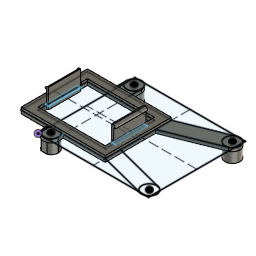
Eris LCD Mount Pi Attachment v2 (Autodesk Fusion 360 design; units mm, degrees)
Autodesk Fusion 360 part; units mm, degrees
sketch "Sketch1" plane through (0, 0, 0) normal (0, 0, 1) x (1, 0, 0)
  line L0 (0, 0) -> (65, 0)
  line L1 (65, 0) -> (65, 57)
  line L2 (65, 57) -> (0, 57)
  line L3 (0, 57) -> (0, 0)
  line L4 (-17, 7) -> (32.5, 7)
  line L5 (32.5, 7) -> (32.5, 46)
  line L6 (32.5, 46) -> (-17, 46)
  line L7 (-17, 46) -> (-17, 7)
  line L8 (7.75, 46) -> (7.75, 7) construction
  line L9 (-17, 26.5) -> (32.5, 26.5) construction
  line L10 (-12, 12) -> (27.5, 12)
  line L11 (27.5, 12) -> (27.5, 41)
  line L12 (27.5, 41) -> (-12, 41)
  line L13 (-12, 41) -> (-12, 12)
  line L14 (-12, 26.5) -> (-11, 26.5) construction
  line L15 (-11, 26.5) -> (-11, 36)
  line L16 (-11, 36) -> (-12, 36)
  line L17 (-12, 36) -> (-12, 26.5) construction
  line L18 (-11, 26.5) -> (-12, 26.5) construction
  line L19 (-12, 26.5) -> (-12, 17) construction
  line L20 (-12, 17) -> (-11, 17)
  line L21 (-11, 17) -> (-11, 26.5)
  line L22 (27.5, 36) -> (26.25, 36)
  line L23 (26.25, 36) -> (26.25, 26.5)
  line L24 (26.25, 26.5) -> (27.5, 26.5) construction
  line L25 (27.5, 26.5) -> (27.5, 36) construction
  line L26 (27.5, 26.5) -> (26.25, 26.5) construction
  line L27 (26.25, 26.5) -> (26.25, 17)
  line L28 (26.25, 17) -> (27.5, 17)
  line L29 (27.5, 17) -> (27.5, 26.5) construction
  line L30 (-12, 36) -> (-13, 36)
  line L31 (-13, 36) -> (-13, 17)
  line L32 (-13, 17) -> (-12, 17)
  line L33 (-12, 17) -> (-12, 36)
  line L34 (27.5, 36) -> (28.5, 36)
  line L35 (28.5, 36) -> (28.5, 17)
  line L36 (28.5, 17) -> (27.5, 17)
  line L37 (27.5, 17) -> (27.5, 36)
  line L38 (32.5, 57) -> (32.5, 0) construction
  line L39 (65, 28.5) -> (0, 28.5) construction
  circle A0 centre (3.5, 53) radius 1.35
  circle A1 centre (61.5, 53) radius 1.35
  circle A2 centre (61.5, 4) radius 1.35
  circle A3 centre (3.5, 4) radius 1.35
  circle A4 centre (3.5, 53) radius 4.35
  circle A5 centre (61.5, 53) radius 4.35
  circle A6 centre (3.5, 4) radius 4.35
  circle A7 centre (61.5, 4) radius 4.35
  line L40 (7.75, 46) -> (7.8496, 52.9376)
  line L41 (-0.8496, 53.0624) -> (-0.9509, 46)
  line L42 (7.8496, 4.0624) -> (7.75, 7)
  line L43 (32.5, 7) -> (60.4118, -0.2117)
  line L44 (32.5, 46) -> (59.8736, 57.0345)
  line L45 (32.5, 15.9857) -> (62.5882, 8.2117)
  line L46 (32.5, 36.6197) -> (63.1264, 48.9655)
  line L47 (-0.85, 4) -> (-0.85, 7)
  dimension "d1" = 65
  dimension "d2" = 57
  dimension "d3" = 17
  dimension "d5" = 49.5
  dimension "d6" = 39
  dimension "d7" = 7
  dimension "d8" = -5
  dimension "d13" = 1
  dimension "d21" = 2.7
  dimension "d22" = 2.7
  dimension "d23" = 2.7
  dimension "d24" = 2.7
  dimension "d26" = 29
  dimension "d27" = 29
  dimension "d28" = 29
  dimension "d29" = 29
  dimension "d30" = 24.5
  dimension "d31" = 24.5
  dimension "d32" = 24.5
  dimension "d33" = 24.5
  dimension "d34" = 3
  dimension "d35" = 3
  dimension "d36" = 3
  dimension "d37" = 3
  constraint horizontal L0
  constraint vertical L1
  constraint horizontal L2
  constraint vertical L3
  constraint coincident L0.start L3.end
  constraint horizontal L4
  constraint vertical L5
  constraint horizontal L6
  constraint vertical L7
  constraint midpoint L6 L8.start
  constraint midpoint L4 L8.end
  constraint midpoint L7 L9.start
  constraint midpoint L5 L9.end
  constraint midpoint L13 L14.start
  constraint coincident L13 L19.end
  constraint horizontal L14
  constraint vertical L15
  constraint horizontal L16
  constraint vertical L17
  constraint horizontal L18
  constraint vertical L19
  constraint horizontal L20
  constraint vertical L21
  constraint horizontal L22
  constraint vertical L23
  constraint horizontal L24
  constraint vertical L25
  constraint horizontal L26
  constraint vertical L27
  constraint horizontal L28
  constraint vertical L29
  constraint horizontal L30
  constraint vertical L31
  constraint horizontal L32
  constraint vertical L33
  constraint horizontal L34
  constraint vertical L35
  constraint horizontal L36
  constraint vertical L37
  constraint midpoint L2 L38.start
  constraint midpoint L0 L38.end
  constraint midpoint L1 L39.start
  constraint midpoint L3 L39.end
  constraint coincident A4 L40.end
  constraint tangent A4 L40
  constraint coincident A4 L41.start
  constraint coincident L6 L41.end
  constraint parallel L40 L41
  constraint coincident A6 L42.start
  constraint coincident A7 L43.end
  constraint tangent A7 L43
  constraint coincident A5 L44.end
  constraint tangent A5 L44
  constraint coincident L5 L45.start
  constraint coincident A7 L45.end
  constraint tangent A7 L45
  constraint coincident L5 L46.start
  constraint coincident A5 L46.end
  constraint tangent A5 L46
  constraint parallel L44 L46
  constraint parallel L43 L45
  constraint tangent A4 L41
  constraint coincident A6 L47.start
  constraint coincident L4 L47.end
  constraint perpendicular L4 L47
  constraint tangent A6 L47
  measures "d1" distance of L0.start L0.end
  measures "d2" distance of L0.start L2.end
  measures "d3" distance of L3 L7
  measures "d5" distance of L4.start L4.end
  measures "d6" distance of L4 L6
  measures "d7" distance of L0 L4
  measures "d13" distance of L22.start L34.end
  measures "d21" diameter of A0
  measures "d22" diameter of A1
  measures "d23" diameter of A2
  measures "d24" diameter of A3
  measures "d26" distance of L38 A0.centre
  measures "d27" distance of L38 A1.centre
  measures "d28" distance of L38 A3.centre
  measures "d29" distance of L38 A2.centre
  measures "d30" distance of L39 A1.centre
  measures "d31" distance of L39 A2.centre
  measures "d32" distance of L39 A0.centre
  measures "d33" distance of L39 A3.centre
extrude "Extrude1" add sketch "Sketch1" along normal blind 1.5 contours L3 L4 L6 L7 L10 L12 L13 L30 L31 L32 | L3 L4 L5 L6 L10 L11 L12 L34 L35 L36 A6 | L4 A6 | L13 L30 L31 L32 L33 | L11 L34 L35 L36 L37 makes body 1
extrude "Extrude2" add sketch "Sketch1" along normal blind 9.3 contours L13 L15 L16 L20 L21 L33 | L11 L22 L23 L27 L28 L37 bodies 1
extrude "Extrude3" add sketch "Sketch1" along normal blind 1.5 from surface at 8.05 contours L13 L30 L31 L32 L33 | L13 L15 L16 L20 L21 L33 | L11 L22 L23 L27 L28 L37 | L11 L34 L35 L36 L37 bodies 1
fillet "Fillet1" radius 1.5 4 edges at (-12, 17, 0.75) (-12, 36, 0.75) (27.5, 17, 0.75) (27.5, 36, 0.75) on bodies 1
fillet "Fillet2" radius 1.5 2 edges at (-13, 26.5, 9.55) (28.5, 26.5, 9.55) on bodies 1
extrude "Extrude4" add sketch "Sketch1" against normal blind 2 separate body contours L0 L3 L4 A6 L42 | L0 A6 | L3 A6 | L3 L4 A6 L47 | L3 L4 A6 | L4 A6 | L4 A6 L42 | L2 L5 A5 L44 L46 | L3 L6 A4 L41 | L3 L6 A4 L40 | L1 L2 A5 | L1 A5 | L3 A4 | L2 L3 A4 | L2 A5 | L2 A4 picked at (64.2833, 53) picked at (0.7167, 53) makes body 2 at (3.3994, 47.8846, 0) makes body 3 at (41.8368, 44.9005, -2) makes body 4 at (0.5946, 5.1952, 0)
extrude "Extrude5" add sketch "Sketch1" against normal up to surface (2 mm away) contours L3 L4 L6 L7 L10 L12 L13 L30 L31 L32 | L3 L4 L5 L6 L10 L11 L12 L34 L35 L36 A6 | L13 L30 L31 L32 L33 | L13 L15 L16 L20 L21 L33 | L11 L22 L23 L27 L28 L37 | L11 L34 L35 L36 L37 bodies 1 2 3 4
extrude "Extrude6" add sketch "Sketch1" against normal blind 6 from surface at -2 separate body contours L0 L3 L4 A6 L42 | L3 A6 | L4 A6 | L1 L2 A5 | L1 A5 | L3 A4 | L2 L3 A4 | L2 A5 | L2 A4 picked at (64.2833, 53) picked at (0.7167, 53) makes body 5 at (3.3916, 48.6514, -4) makes body 6 at (65.8284, 52.5669, -6) makes body 7 at (7.8004, 4.6553, -4)
equation "d5 = 39.5 mm + 10 mm"
equation "d6 = 29 mm + 10 mm"
equation "d11 = 3 mm + 6.3 mm"
equation "d14 = 6.3 mm + 1.5 mm + 0.25 mm"
equation "d26 = ( 58 / 2 ) * 1 mm"
equation "d27 = ( 58 / 2 ) * 1 mm"
equation "d28 = ( 58 / 2 ) * 1 mm"
equation "d29 = ( 58 / 2 ) * 1 mm"
equation "d30 = ( 49 / 2 ) * 1 mm"
equation "d31 = ( 49 / 2 ) * 1 mm"
equation "d32 = ( 49 / 2 ) * 1 mm"
